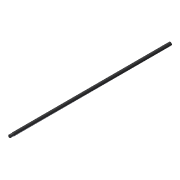
# Autodesk Inventor part: Pipe1
Saved by Autodesk Inventor 2014 SP1 (Build 180222100, 222)
## iProperties
Created: 2014-12-05
Part Number: Pipe1
Material: Generic
Document SubType Name: Modeling
Designer: AlecShufelt
Density: 1 g/cm^3
Appearance: Dark Gray
Author: AlecShufelt
Autodesk Inventor part; units mm, degrees
ref_plane "YZ Plane" through (0, 0, 0) normal (1, 0, 0) x (0, 1, 0)
ref_plane "XZ Plane" through (0, 0, 0) normal (0, 1, 0) x (-1, 0, 0)
ref_plane "XY Plane" through (0, 0, 0) normal (0, 0, 1) x (1, 0, 0)
sketch "Sketch1" plane through (0, 0, 0) normal (0, 0, 1) x (1, 0, 0)
  circle A0 centre (0, 0) radius 7.4168
  circle A1 centre (0, 0) radius 10.8839
  dimension "d0" = 14.8336
  dimension "d1" = 21.7678
  constraints: 2 centre point, 2 coincident
  measures "d0" diameter of A0
  measures "d1" diameter of A1
extrude "Extrusion1" add sketch "Sketch1" along normal blind 1128.3188
sketch "Sketch2" plane through (0, 0, 1128.3188) normal (0, 0, 1) x (1, 0, 0)
  circle A0 centre (0, 0) radius 10.8839 projected
  circle A1 centre (0, 0) radius 9.662
  constraints: 1 centre point, 1 coincident
extrude "Extrusion2" cut sketch "Sketch2" against normal blind 25.4
thread "Thread2" size "13/16-10 UNC" class "2A" standard "ANSI Unified Screw Threads" full length
body "Solid1"
